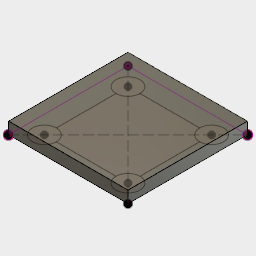
C03-W2-PE-01 (Autodesk Fusion 360 design; units mm, degrees)
Autodesk Fusion 360 part; units mm, degrees
sketch "Sketch1" plane through (0, 0, 0) normal (0, 1, 0) x (1, 0, 0)
  line L0 (-50, 50) -> (50, 50)
  line L1 (50, 50) -> (50, -50)
  line L2 (50, -50) -> (-50, -50)
  line L3 (-50, -50) -> (-50, 50)
  line L4 (-50, 50) -> (50, -50) construction
  line L5 (50, 50) -> (-50, -50) construction
  dimension "d1" = 100
  dimension "d2" = 100
  measures "d1" distance of L0.end L1.end
  measures "d2" distance of L1.end L2.end
extrude "Extrude1" add sketch "Sketch1" along normal blind 10
sketch "CUT" plane through (0, 0, 0) normal (0, 1, 0) x (1, 0, 0)
  line L0 (-50, 50) -> (50, -50) construction
  line L1 (-50, -50) -> (50, 50) construction
  circle A0 centre (-35, 35) radius 10
  circle A1 centre (35, 35) radius 10
  circle A2 centre (35, -35) radius 10
  circle A3 centre (-35, -35) radius 10
  line L2 (50, 50) -> (-50, 50)
  line L3 (-50, 50) -> (-50, -50)
  line L4 (-25, 35) -> (25, 35)
  line L5 (25, -35) -> (-25, -35)
  line L6 (-35, 25) -> (-35, -25)
  line L7 (35, -25) -> (35, 25)
  point P0 (-50, 50)
  point P1 (50, -50)
  point P2 (-50, -50)
  point P3 (50, 50)
  dimension "d5" = 20
  dimension "d6" = 15
  measures "d5" diameter of A0
  measures "d6" distance of A0.centre L2
named bodies: "BODY"
